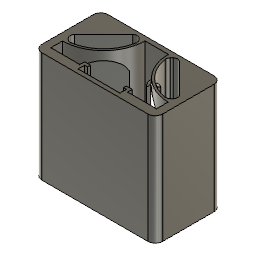
Imaging_Enclosure (Autodesk Fusion 360 design; units mm, degrees)
part number: 2026-03-22-21-42-42-827
Autodesk Fusion 360 part; units mm, degrees
note: some values were not read from the file. Set by a fixed rule: which face or edge a step refers to.
sketch "Sketch1" plane through (0, 0, 0) normal (0, 0, 1) x (1, 0, 0)
  line L0 (-43.0895, 22.8761) -> (56.9105, 22.8761)
  line L1 (56.9105, 22.8761) -> (56.9105, -20.1239)
  line L2 (56.9105, -20.1239) -> (-43.0895, -20.1239)
  line L3 (-43.0895, -20.1239) -> (-43.0895, 22.8761)
  dimension "d1" = 100
  dimension "d2" = 43
  constraint horizontal L0
  constraint vertical L1
  constraint horizontal L2
  constraint vertical L3
  measures "d1" distance of L0.start L0.end
  measures "d2" distance of L0.start L2.end
extrude "Extrude1" add sketch "Sketch1" along normal blind 75 makes body 1
sketch "TOP" plane through (0, 0, 75) normal (0, 0, 1) x (-1, 0, 0)
  line L0 (43.0895, 20.1239) -> (-56.9105, 20.1239)
  line L1 (-56.9105, 20.1239) -> (-56.9105, -22.8761)
  line L2 (-56.9105, -22.8761) -> (43.0895, -22.8761)
  line L3 (43.0895, -22.8761) -> (43.0895, 20.1239)
  line L4 (39.0895, -19.8761) -> (-52.9105, -19.8761)
  line L5 (-52.9105, -19.8761) -> (-52.9105, 16.1239)
  line L6 (-52.9105, 16.1239) -> (39.0895, 16.1239)
  line L7 (39.0895, 16.1239) -> (39.0895, -19.8761)
  line L8 (-6.9105, 16.1239) -> (-6.9105, 19.1239)
  line L9 (-6.9105, 16.1239) -> (16.0704, -6.8571)
  line L10 (-6.9105, 16.1239) -> (25.5895, 16.1239) construction
  line L11 (-6.9105, 16.1239) -> (-32.3664, -9.332)
  line L12 (-6.9105, 16.1239) -> (29.0895, 16.1239) construction
  line L13 (-32.3664, -9.332) -> (-21.8222, -19.8761)
  line L14 (-32.3664, -9.332) -> (-17.4547, -9.332) construction
  line L15 (-32.3664, -9.332) -> (-52.9105, 11.2122)
  line L16 (16.0704, -6.8571) -> (3.0514, -19.8761)
  line L17 (16.0704, -6.8571) -> (39.0895, 16.1619)
  line L18 (16.0704, -6.8571) -> (48.6243, -6.8571) construction
  line L19 (-32.3664, -9.332) -> (-44.2281, 2.5297)
  line L20 (-32.3664, -9.332) -> (-15.5914, -9.332) construction
  line L21 (-32.3664, -9.332) -> (-20.5047, -21.1937)
  line L22 (-20.5047, -21.1937) -> (-16.501, -17.1901)
  line L23 (-20.5047, -21.1937) -> (-14.8427, -21.1937) construction
  line L24 (-44.2281, 2.5297) -> (-40.2245, 6.5334)
  line L25 (-32.3664, -9.332) -> (-24.1993, -1.1649)
  line L26 (-20.5047, -21.1937) -> (-19.0904, -19.7795)
  line L27 (-19.0904, -19.7795) -> (-16.3404, -19.7795)
  line L28 (-44.2281, 2.5297) -> (-42.8139, 3.9439)
  line L29 (-42.8139, 3.9439) -> (-42.8139, 6.6939)
  arc A0 (-16.3404, -19.7795) -> (-42.8139, 6.6939) centre (-43.1782, -20.1438) ccw
  line L30 (-24.1993, -1.1649) -> (-23.1386, -0.1042)
  line L31 (-16.3404, -19.7795) -> (-14.8404, -19.7795)
  line L32 (-42.8139, 6.6939) -> (-42.8139, 8.1939)
  line L33 (-42.8139, 8.1939) -> (-42.8139, 16.1239)
  arc A1 (-14.8404, -19.7795) -> (-42.8139, 8.1939) centre (-43.1779, -20.1435) ccw
  line L34 (-6.9105, 16.1239) -> (-6.9105, -19.8761)
  line L35 (-16.501, -17.1901) -> (-20.5047, -21.1937)
  line L36 (-40.2245, 6.5334) -> (-44.2281, 2.5297)
  line L37 (-40.2245, 6.5334) -> (-44.2281, 2.5297)
  line L38 (-42.8139, 3.9439) -> (-40.2245, 6.5334)
  line L39 (-19.1871, -19.8761) -> (-16.501, -17.1901)
  line L40 (-24.1993, -1.1649) -> (-32.6492, -9.6148)
  line L41 (-32.6492, -9.6148) -> (-20.6461, -21.618)
  line L42 (-32.6492, -9.6148) -> (-15.6742, -9.6148) construction
  line L43 (-20.6461, -21.618) -> (-16.4739, -17.4458)
  line L44 (-32.6492, -9.6148) -> (-44.6524, 2.3883)
  line L45 (-32.6492, -9.6148) -> (-15.6742, -9.6148) construction
  line L46 (-44.6524, 2.3883) -> (-40.4802, 6.5605)
  line L47 (-14.8404, -19.7795) -> (-14.8404, -19.8761)
  line L48 (7.2891, 14.9239) -> (-21.1109, 14.9239)
  line L49 (-21.1109, 14.9239) -> (-21.1109, 19.3239)
  line L50 (-21.1109, 19.3239) -> (7.2891, 19.3239)
  line L51 (7.2891, 19.3239) -> (7.2891, 14.9239)
  line L52 (-6.9105, 16.1239) -> (0.1895, 16.1239)
  dimension "d5" = 92
  dimension "d6" = 36
  dimension "d7" = 4
  dimension "d8" = 3
  dimension "d9" = 3
  dimension "d10" = 46
  dimension "d11" = 32.5
  dimension "d12" = 45
  dimension "d13" = 135
  dimension "d14" = 36
  dimension "d15" = 45
  dimension "d16" = 45
  dimension "d17" = 135
  dimension "d18" = 16.775
  dimension "d19" = 16.775
  dimension "d20" = 45
  dimension "d21" = 5.662
  dimension "d22" = 5.662
  dimension "d23" = 11.55
  dimension "d24" = 2
  dimension "d25" = 2.75
  dimension "d26" = 2
  dimension "d27" = 2.75
  dimension "d28" = 1.5
  dimension "d29" = 1.5
  dimension "d30" = 1.5
  dimension "d31" = 11.95
  dimension "d32" = 45
  dimension "d33" = 16.975
  dimension "d34" = 135
  dimension "d35" = 16.975
  dimension "d105" = 28.4
  dimension "d106" = 4.4
  dimension "d107" = 1.2
  dimension "d108" = 21.703
  dimension "d124" = 7.1
  constraint horizontal L4
  constraint vertical L5
  constraint horizontal L6
  constraint vertical L7
  constraint coincident L6 L8.start
  constraint perpendicular L6 L8
  constraint horizontal L10
  constraint horizontal L12
  constraint horizontal L14
  constraint coincident L4 L13.end
  constraint coincident L5 L15.end
  constraint perpendicular L11 L15
  constraint coincident L4 L16.end
  constraint perpendicular L9 L16
  constraint horizontal L18
  constraint coincident L7 L17.end
  constraint horizontal L20
  constraint perpendicular L11 L21
  constraint horizontal L23
  constraint perpendicular L19 L24
  constraint perpendicular L13 L25
  constraint perpendicular L21 L26
  constraint horizontal L27
  constraint perpendicular L19 L28
  constraint vertical L29
  constraint coincident L25.end A0
  constraint parallel L11 L30
  constraint parallel L27 L31
  constraint parallel L29 L32
  constraint vertical L33
  constraint coincident L6 L33.end
  constraint coincident L30.end A1
  constraint midpoint L4 L34.end
  constraint coincident L4 L39.start
  constraint coincident L26 L39.start
  constraint parallel L25 L40
  constraint horizontal L42
  constraint coincident A0 L43.end
  constraint perpendicular L41 L43
  constraint horizontal L45
  constraint coincident A0 L46.end
  constraint perpendicular L44 L46
  constraint vertical L47
  constraint coincident L4 L47.end
  constraint horizontal L48
  constraint vertical L49
  constraint horizontal L50
  constraint vertical L51
  constraint perpendicular L51 L52
  measures "d5" distance of L4.start L4.end
  measures "d6" distance of L4.start L6.end
  measures "d7" distance of L1 L5
  measures "d8" distance of L2 L4
  measures "d9" distance of L8.start L8.end
  measures "d10" distance of L5 L8
  measures "d11" distance of L8.start L9.end
  measures "d12" angle of L9 L10
  measures "d13" angle of L11 L12
  measures "d14" distance of L8.start L11.end
  measures "d15" angle of L13 L14
  measures "d16" angle of L17 L18
  measures "d17" angle of L19 L20
  measures "d18" distance of L11.end L19.end
  measures "d19" distance of L11.end L21.end
  measures "d20" angle of L22 L23
  measures "d21" distance of L21.end L22.end
  measures "d22" distance of L19.end L24.end
  measures "d23" distance of L11.end L25.end
  measures "d24" distance of L21.end L26.end
  measures "d25" distance of L26.end L27.end
  measures "d26" distance of L19.end L28.end
  measures "d27" distance of L28.end L29.end
  measures "d28" distance of L25.end L30.end
  measures "d29" distance of L27.end L31.end
  measures "d30" distance of L29.end L32.end
  measures "d31" distance of L25.end L40.end
  measures "d32" angle of L41 L42
  measures "d33" distance of L40.end L41.end
  measures "d34" angle of L44 L45
  measures "d35" distance of L40.end L44.end
  measures "d105" distance of L48.start L48.end
  measures "d106" distance of L48.start L50.end
  measures "d107" distance of L12 L48
  measures "d108" distance of L33 L49
  measures "d124" distance of L8.start L52.end
sketch "Sketch3" plane through (0, -20.1239, 0) normal (0, -1, 0) x (1, 0, 0)
  line L0 (-43.0895, 0) -> (56.9105, 0)
  line L1 (56.9105, 0) -> (56.9105, 75)
  line L2 (56.9105, 75) -> (-43.0895, 75)
  line L3 (-43.0895, 75) -> (-43.0895, 0)
extrude "Extrude2" cut sketch "TOP" against normal blind 41.25 contours L4 L21 L22 L26 L35 L41 L43 | L4 L22 L26 L27 L35 L39 L43 | L4 L21 L22 L26 L35 | L4 L11 L13 L21 L22 L25 L26 A0 L35 L39 L40 | L22 L27 A0 L35 L39 L43 | L4 L13 L21 L40 L41 | L11 L15 L19 L24 L25 L28 A0 L36 L37 L38 L40 | L15 L19 L40 L44 L46 | L24 L29 A0 L36 L37 L38 L46 | L15 L24 L28 L29 L36 L37 L46 bodies 1
extrude "Extrude3" cut sketch "TOP" against normal blind 51.25 contours L4 L21 L22 L26 L35 L41 L43 | L4 L22 L26 L27 L35 L39 L43 | L4 L21 L22 L26 L35 | L4 L11 L13 L21 L22 L25 L26 A0 L35 L39 L40 | L22 L27 A0 L35 L39 L43 | L4 L13 L21 L40 L41 | L11 L15 L19 L24 L25 L28 A0 L36 L37 L38 L40 | L15 L19 L40 L44 L46 | L24 L29 A0 L36 L37 L38 L46 | L15 L24 L28 L29 L36 L37 L46 bodies 1
extrude "Extrude4" cut sketch "TOP" against normal blind 71 contours L4 L9 L16 L34 L48 | L4 L11 A1 L34 L47 L48 | L6 L9 L17 L48 L51 | L11 L34 L48 | L9 L34 L48 | L6 L9 L48 L51 L52 | L6 L11 L48 L49 | L6 L11 L33 A1 L48 L49 bodies 1
sketch "Sketch4" plane through (21.132, 21.132, 0) normal (-0.707107, -0.707107, 0) x (0.707107, -0.707107, 0)
  line L0 (33.2628, 75) -> (-0.6872, 75)
  line L1 (-0.6872, 75) -> (-0.6872, 23.75)
  line L2 (-0.6872, 23.75) -> (33.2628, 23.75)
  line L3 (33.2628, 23.75) -> (33.2628, 75)
  line L4 (3.9498, 60.75) -> (28.6258, 60.75)
  line L5 (28.6258, 60.75) -> (28.6258, 27.75)
  line L6 (28.6258, 27.75) -> (3.9498, 27.75)
  line L7 (3.9498, 27.75) -> (3.9498, 60.75)
  line L8 (3.9498, 54.2255) -> (16.2878, 54.2255) construction
  line L9 (16.2878, 54.2255) -> (16.2878, 27.75) construction
  line L10 (16.2878, 54.2255) -> (16.2878, 68.7495) construction
  arc A0 (28.6258, 60.75) -> (3.9498, 60.75) centre (16.2878, 55.2351) ccw construction
  dimension "d42" = 24.676
  dimension "d43" = 33
  dimension "d44" = 4.637
  dimension "d45" = 4
  dimension "d46" = 12.338
  dimension "d47" = 14.524
  constraint horizontal L4
  constraint vertical L5
  constraint horizontal L6
  constraint vertical L7
  constraint coincident L7 L8.start
  constraint perpendicular L7 L8
  constraint midpoint L6 L9.end
  constraint perpendicular L8 L10
  constraint coincident L10.end A0
  measures "d42" distance of L4.start L4.end
  measures "d43" distance of L4.start L6.end
  measures "d44" distance of L1 L7
  measures "d45" distance of L2 L6
  measures "d46" distance of L8.start L8.end
  measures "d47" distance of L8.end L10.end
sketch "Sketch5" plane through (21.132, 21.132, 0) normal (-0.707107, -0.707107, 0) x (0.707107, -0.707107, 0)
  line L0 (33.2628, 75) -> (-0.6872, 75)
  line L1 (-0.6872, 75) -> (-0.6872, 23.75)
  line L2 (-0.6872, 23.75) -> (33.2628, 23.75)
  line L3 (33.2628, 23.75) -> (33.2628, 75)
  line L4 (3.9498, 61.1) -> (28.6258, 61.1)
  line L5 (28.6258, 61.1) -> (28.6258, 28.1)
  line L6 (28.6258, 28.1) -> (3.9498, 28.1)
  line L7 (3.9498, 28.1) -> (3.9498, 61.1)
  line L8 (16.2878, 28.1) -> (16.2878, 69.1)
  arc A0 (28.6258, 61.1) -> (3.9498, 61.1) centre (16.2878, 55.5859) ccw
  dimension "d48" = 24.676
  dimension "d49" = 33
  dimension "d50" = 4.637
  dimension "d51" = 4.35
  dimension "d52" = 41
  constraint horizontal L4
  constraint vertical L5
  constraint horizontal L6
  constraint vertical L7
  constraint vertical L8
  constraint midpoint L6 L8.start
  constraint coincident L8.end A0
  measures "d48" distance of L4.start L4.end
  measures "d49" distance of L4.start L6.end
  measures "d50" distance of L1 L7
  measures "d51" distance of L2 L6
  measures "d52" distance of L8.start L8.end
extrude "Extrude5" cut sketch "Sketch5" along normal blind 14 contours L4 L8 A0 | L4 L6 L7 L8 | L4 L8 A0 | L4 L5 L6 L8 bodies 1
fillet "Fillet1" radius 3 4 edges at (20.6461, 21.618, 49.375) (16.4739, 17.4458, 49.375) (40.4802, -6.5605, 49.375) (44.6524, -2.3883, 49.375) on bodies 1
sketch "Sketch6" plane through (0, 22.8761, 0) normal (0, 1, 0) x (-1, 0, 0)
  line L0 (-56.9105, 0) -> (43.0895, 0)
  line L1 (43.0895, 0) -> (43.0895, 75)
  line L2 (43.0895, 75) -> (-56.9105, 75)
  line L3 (-56.9105, 75) -> (-56.9105, 0)
  line L4 (-6.9105, 0) -> (-6.9105, 75)
  line L5 (43.0895, 7.2495) -> (-56.9105, 7.2495)
  circle A0 centre (-6.9105, 35.85) radius 7
  circle A1 centre (-6.9105, 48.35) radius 7
  line L6 (3.5895, 23.35) -> (-17.4105, 23.35)
  line L7 (-17.4105, 23.35) -> (-17.4105, 35.85)
  line L8 (-17.4105, 35.85) -> (3.5895, 35.85)
  line L9 (3.5895, 35.85) -> (3.5895, 23.35)
  line L10 (3.5895, 35.85) -> (-17.4105, 35.85)
  line L11 (-17.4105, 35.85) -> (-17.4105, 48.35)
  line L12 (-17.4105, 48.35) -> (3.5895, 48.35)
  line L13 (3.5895, 48.35) -> (3.5895, 35.85)
  line L14 (3.5895, 29.6) -> (-17.4105, 29.6)
  line L15 (-17.4105, 29.6) -> (-17.4105, 42.1)
  line L16 (-17.4105, 42.1) -> (3.5895, 42.1)
  line L17 (3.5895, 42.1) -> (3.5895, 29.6)
  line L18 (0.0895, 48.35) -> (0.0895, 35.85)
  line L19 (-13.9105, 35.85) -> (-13.9105, 48.35)
  line L20 (-2.5605, 22.65) -> (-11.2605, 22.65)
  line L21 (-11.2605, 22.65) -> (-11.2605, 34.65)
  line L22 (-11.2605, 34.65) -> (-2.5605, 34.65)
  line L23 (-2.5605, 34.65) -> (-2.5605, 22.65)
  circle A2 centre (3.5895, 23.35) radius 0.85
  circle A3 centre (3.5895, 29.6) radius 0.85
  circle A4 centre (3.5895, 35.85) radius 0.85
  circle A5 centre (3.5895, 42.1) radius 0.85
  circle A6 centre (3.5895, 48.35) radius 0.85
  circle A7 centre (-17.4105, 48.35) radius 0.85
  circle A8 centre (-17.4105, 42.1) radius 0.85
  circle A9 centre (-17.4105, 35.85) radius 0.85
  circle A10 centre (-17.4105, 29.6) radius 0.85
  circle A11 centre (-17.4105, 23.35) radius 0.85
  dimension "d57" = 50
  dimension "d58" = 14
  dimension "d59" = 50
  dimension "d60" = 35.85
  dimension "d61" = 14
  dimension "d62" = 48.35
  dimension "d72" = 21
  dimension "d73" = 12.5
  dimension "d74" = 12.5
  dimension "d75" = 10.5
  dimension "d76" = 21
  dimension "d77" = 12.5
  dimension "d78" = 12.5
  dimension "d79" = 10.5
  dimension "d80" = 21
  dimension "d81" = 12.5
  dimension "d82" = 6.25
  dimension "d83" = 8.7
  dimension "d84" = 12
  dimension "d85" = 0.7
  dimension "d86" = 4.35
  dimension "d87" = 1.7
  dimension "d88" = 1.7
  dimension "d89" = 1.7
  dimension "d90" = 1.7
  dimension "d91" = 1.7
  dimension "d92" = 1.7
  dimension "d93" = 1.7
  dimension "d94" = 1.7
  dimension "d95" = 1.7
  dimension "d96" = 1.7
  constraint coincident L0 L4.start
  constraint coincident L2 L4.end
  constraint perpendicular L2 L4
  constraint coincident L1 L5.start
  constraint coincident L3 L5.end
  constraint perpendicular L3 L5
  constraint coincident L4 A1.centre
  constraint horizontal L6
  constraint vertical L7
  constraint horizontal L8
  constraint vertical L9
  constraint horizontal L10
  constraint vertical L11
  constraint horizontal L12
  constraint vertical L13
  constraint horizontal L14
  constraint vertical L15
  constraint horizontal L16
  constraint vertical L17
  constraint coincident L9 L14.start
  constraint coincident L12 L18.start
  constraint coincident A1 L18.start
  constraint coincident L10 L18.end
  constraint coincident A0 L18.end
  constraint coincident A0 L19.start
  constraint coincident L8 L19.start
  constraint coincident A1 L19.end
  constraint coincident L12 L19.end
  constraint horizontal L20
  constraint vertical L21
  constraint horizontal L22
  constraint vertical L23
  constraint coincident L6.start L9.end
  constraint coincident L14.start L17.end
  constraint coincident L8.end L9.start
  constraint coincident L16.end L17.start
  constraint coincident L12.end L13.start
  constraint coincident L11.end L12.start
  constraint coincident L15.end L16.start
  constraint coincident L7.end L8.start
  constraint coincident L14.end L15.start
  constraint coincident L6.end L7.start
  measures "d57" distance of L3 L4
  measures "d58" diameter of A0
  measures "d59" distance of L3 A0.centre
  measures "d60" distance of L0 A0.centre
  measures "d61" diameter of A1
  measures "d62" distance of L0 A1.centre
  measures "d72" distance of L6.start L6.end
  measures "d73" distance of L6.start L8.end
  measures "d74" distance of A0.centre L6
  measures "d75" distance of A0.centre L7
  measures "d76" distance of L8.end L7.end
  measures "d77" distance of L8.end L12.end
  measures "d78" distance of A1.centre L10
  measures "d79" distance of A1.centre L11
  measures "d80" distance of L14.start L14.end
  measures "d81" distance of L14.start L16.end
  measures "d82" distance of L12 L16
  measures "d83" distance of L20.start L20.end
  measures "d84" distance of L20.start L22.end
  measures "d85" distance of L6 L20
  measures "d86" distance of L4 L21
  measures "d87" diameter of A2
  measures "d88" diameter of A3
  measures "d89" diameter of A4
  measures "d90" diameter of A5
  measures "d91" diameter of A6
  measures "d92" diameter of A7
  measures "d93" diameter of A8
  measures "d94" diameter of A9
  measures "d95" diameter of A10
  measures "d96" diameter of A11
extrude "Extrude6" add 1 faces at (17.6517, 10.4832, 28.1) along direction (0, 0, 1) blind 45 on bodies 1 bodies 1
extrude "Extrude7" add 1 faces at (29.408, 7.2534, 23.75) along direction (0, 0, 1) blind 0.35 on bodies 1 bodies 1
extrude "Extrude8" cut sketch "Sketch5" along normal blind 15 contours L4 L8 A0 | L4 L6 L7 L8 | L4 L8 A0 | L4 L5 L6 L8 bodies 1
sketch "Sketch7" plane through (0, 0, 0) normal (0, 1, 0) x (1, 0, 0)
extrude "Extrude9" cut sketch "Sketch6" against normal blind 2.5 contours L6 L9 A2 | L6 L9 A2 | L6 L7 A11 | L6 L7 A11 | L12 L13 A6 | L12 L13 A6 | L11 L12 A7 | L11 L12 A7 | L9 L14 L17 A3 | L9 L14 A3 | L7 L14 A10 | L7 L14 L15 A10 | L13 L16 A5 | L13 L16 L17 A5 | L11 L15 L16 A8 | L11 L16 A8 | L9 L17 A3 | L7 L15 A10 | L8 L10 L13 L17 A4 | L8 L9 L10 L17 A4 | L13 L17 A5 | L7 L8 L10 L15 A9 | L8 L10 L11 L15 A9 | L11 L15 A8 | L9 L13 L17 A4 | L7 L11 L15 A9 bodies 1
extrude "Extrude10" cut sketch "Sketch6" against normal blind 3 contours L4 L6 L20 L21 | L4 L6 L20 L23 | L4 A0 L6 L14 L21 | L4 A0 L6 L14 L23 | L4 A1 L12 | L4 A1 L12 | L4 A0 L14 | L4 A0 L14 | L4 A0 A1 L12 | L4 A0 A1 L12 | A1 L16 L18 | A1 L16 L19 | L4 A0 L14 L21 L22 | L4 A0 L14 L22 L23 | A0 L14 L21 | A0 L14 L23 | L4 A0 L16 | L4 A0 L16 | A0 L16 L18 | L4 A0 A1 L8 L10 | L4 A1 L16 | L4 A0 A1 L8 L10 | L4 A1 L16 | A0 L16 L19 | L4 A0 L8 L10 L21 L22 | L4 A0 L8 L10 L22 L23 bodies 1
sketch "Sketch8" plane through (0, 0, 4) normal (0, 0, 1) x (-1, 0, 0)
  arc A0 (-14.8404, -19.7795) -> (-42.8139, 8.1939) centre (-43.1779, -20.1435) ccw
  line L0 (-14.8404, -19.7795) -> (-14.8404, -19.8761)
  line L1 (-14.8404, -19.8761) -> (3.0514, -19.8761)
  line L2 (3.0514, -19.8761) -> (39.0514, 16.1239)
  line L3 (39.0514, 16.1239) -> (-42.8139, 16.1239)
  line L4 (-42.8139, 16.1239) -> (-42.8139, 8.1939)
  line L5 (7.2891, 14.9239) -> (-21.1109, 14.9239)
  line L6 (-21.1109, 14.9239) -> (-21.1109, 19.3239)
  line L7 (-21.1109, 19.3239) -> (7.2891, 19.3239)
  line L8 (7.2891, 19.3239) -> (7.2891, 14.9239)
  dimension "d101" = 28.4
  dimension "d102" = 4.4
  dimension "d103" = 1.2
  dimension "d104" = 21.703
  constraint horizontal L5
  constraint vertical L6
  constraint horizontal L7
  constraint vertical L8
  measures "d101" distance of L5.start L5.end
  measures "d102" distance of L5.start L7.end
  measures "d103" distance of L3 L5
  measures "d104" distance of L4 L6
extrude "Extrude11" cut sketch "TOP" against normal blind 75 contours L11 L34 L48 | L9 L34 L48 | L6 L9 L48 L51 L52 | L6 L49 L50 L51 L52 | L6 L11 L48 L49 bodies 1
extrude "Extrude12" add 1 faces at (23.5772, -20.1239, 25) along direction (0, -1, 0) blind 2 on bodies 1 bodies 1
sketch "Sketch9" plane through (0, 0, 75) normal (0, 0, 1) x (-1, 0, 0)
  line L0 (-56.9105, 22.1239) -> (-56.9105, -22.8761)
  line L1 (-56.9105, -22.8761) -> (43.0895, -22.8761)
  line L2 (43.0895, -22.8761) -> (43.0895, 22.1239)
  line L3 (43.0895, 22.1239) -> (-56.9105, 22.1239)
  line L4 (-17.5175, -18.4894) -> (-18.5248, -19.4967)
  arc A0 (-22.7674, -19.4967) -> (-18.5248, -19.4967) centre (-20.6461, -17.3753) ccw
  line L5 (-22.7674, -19.4967) -> (-42.531, 0.267)
  arc A1 (-42.531, 4.5096) -> (-42.531, 0.267) centre (-40.4097, 2.3883) ccw
  line L6 (-42.531, 4.5096) -> (-41.5238, 5.5168)
  arc A2 (-38.9274, 6.3577) -> (-41.5238, 5.5168) centre (-39.4025, 3.3955) ccw
  arc A3 (-16.6767, -15.893) -> (-38.9274, 6.3577) centre (-43.1782, -20.1438) ccw
  arc A4 (-17.5175, -18.4894) -> (-16.6767, -15.893) centre (-19.6389, -16.3681) ccw
  line L7 (-21.1109, 16.1239) -> (-21.1109, 19.3239)
  line L8 (-21.1109, 19.3239) -> (7.2891, 19.3239)
  line L9 (7.2891, 19.3239) -> (7.2891, 16.1239)
  line L10 (7.2891, 16.1239) -> (39.0514, 16.1239)
  line L11 (39.0514, 16.1239) -> (3.0514, -19.8761)
  line L12 (3.0514, -19.8761) -> (-14.8404, -19.8761)
  line L13 (-14.8404, -19.8761) -> (-14.8404, -19.7795)
  arc A5 (-14.8404, -19.7795) -> (-42.8139, 8.1939) centre (-43.1779, -20.1435) ccw
  line L14 (-42.8139, 8.1939) -> (-42.8139, 16.1239)
  line L15 (-42.8139, 16.1239) -> (-21.1109, 16.1239)
  line L16 (20.0558, 22.1239) -> (-47.9442, 22.1239)
  line L17 (-47.9442, 22.1239) -> (-47.9442, -22.8761)
  line L18 (-47.9442, -22.8761) -> (20.0558, -22.8761)
  line L19 (20.0558, -22.8761) -> (20.0558, 22.1239)
  line L20 (20.0558, 22.1239) -> (23.0558, 22.1239)
  line L21 (23.0558, 22.1239) -> (23.0558, -22.8761)
  dimension "d113" = 68
  dimension "d116" = 3
  constraint horizontal L16
  constraint vertical L17
  constraint horizontal L18
  constraint vertical L19
  constraint coincident L3 L16.start
  constraint perpendicular L19 L20
  constraint coincident L1 L21.end
  constraint perpendicular L1 L21
  measures "d113" distance of L16.start L16.end
  measures "d116" distance of L16.start L20.end
extrude "Extrude13" cut sketch "Sketch9" against normal blind 75 contours L0 L1 L3 L17 bodies 1
extrude "Extrude14" add sketch "Sketch9" against normal blind 75 contours L3 L10 L19 L20 L21 | L1 L11 L19 L21 | L10 L11 L19 L21 bodies 1
extrude "Extrude15" cut sketch "Sketch9" against normal blind 75 contours L1 L2 L3 L10 L11 L21 | L10 L11 L21 bodies 1
sketch "Sketch10" plane through (0, -14.9239, 0) normal (0, -1, 0) x (1, 0, 0)
  line L0 (21.1109, 4) -> (-7.2891, 4)
  line L1 (-7.2891, 4) -> (-7.2891, 0)
  line L2 (-7.2891, 0) -> (21.1109, 0)
  line L3 (21.1109, 0) -> (21.1109, 4)
chamfer "Chamfer1" distance 4 angle 45 1 edges at (6.9109, -14.9239, 0) on bodies 1
sketch "Sketch11" plane through (0, 22.8761, 0) normal (0, 1, 0) x (-1, 0, 0)
  arc A0 (-2.5605, 30.3657) -> (0.0895, 35.85) centre (-6.9105, 35.85) ccw
  line L0 (-2.5605, 30.3657) -> (-2.5605, 22.65)
  line L1 (-2.5605, 22.65) -> (-11.2605, 22.65)
  line L2 (-11.2605, 22.65) -> (-11.2605, 30.3657)
  arc A1 (-13.9105, 35.85) -> (-11.2605, 30.3657) centre (-6.9105, 35.85) ccw
  line L3 (-13.9105, 35.85) -> (-13.9105, 48.35)
  arc A2 (0.0895, 48.35) -> (-13.9105, 48.35) centre (-6.9105, 48.35) ccw
  line L4 (0.0895, 48.35) -> (0.0895, 35.85)
  circle A3 centre (3.5895, 29.6) radius 0.85
  circle A4 centre (-17.4105, 48.35) radius 0.85
  circle A5 centre (-17.4105, 29.6) radius 0.85
  circle A6 centre (3.5895, 48.35) radius 0.85
  circle A7 centre (3.5895, 23.35) radius 0.85
  circle A8 centre (3.5895, 35.85) radius 0.85
  circle A9 centre (-17.4105, 42.1) radius 0.85
  circle A10 centre (-17.4105, 35.85) radius 0.85
  circle A11 centre (3.5895, 42.1) radius 0.85
  circle A12 centre (-17.4105, 23.35) radius 0.85
  line L5 (23.0558, 75) -> (-47.9442, 75)
  line L6 (-47.9442, 0) -> (23.0558, 0)
  line L7 (23.0558, 0) -> (23.0558, 75)
  line L8 (-47.9442, 75) -> (-47.9442, 0)
sketch "Sketch12" plane through (0, 0, 75) normal (0, 0, 1) x (-1, 0, 0)
  line L0 (-48, 22) -> (-7, 22)
  constraint horizontal L0
sketch "Sketch13" plane through (0, 0, 75) normal (0, 0, 1) x (-1, 0, 0)
  line L0 (-17.5175, -18.4894) -> (-18.5248, -19.4967)
  arc A0 (-22.7674, -19.4967) -> (-18.5248, -19.4967) centre (-20.6461, -17.3753) ccw
  line L1 (-22.7674, -19.4967) -> (-42.531, 0.267)
  arc A1 (-42.531, 4.5096) -> (-42.531, 0.267) centre (-40.4097, 2.3883) ccw
  line L2 (-42.531, 4.5096) -> (-41.5238, 5.5168)
  arc A2 (-38.9274, 6.3577) -> (-41.5238, 5.5168) centre (-39.4025, 3.3955) ccw
  arc A3 (-16.6767, -15.893) -> (-38.9274, 6.3577) centre (-43.1782, -20.1438) ccw
  arc A4 (-17.5175, -18.4894) -> (-16.6767, -15.893) centre (-19.6389, -16.3681) ccw
  line L3 (20.0558, 16.1239) -> (20.0558, -2.8718)
  line L4 (20.0558, -2.8718) -> (3.0514, -19.8761)
  line L5 (3.0514, -19.8761) -> (-14.8404, -19.8761)
  line L6 (-14.8404, -19.8761) -> (-14.8404, -19.7795)
  arc A5 (-14.8404, -19.7795) -> (-42.8139, 8.1939) centre (-43.1779, -20.1435) ccw
  line L7 (-42.8139, 8.1939) -> (-42.8139, 16.1239)
  line L8 (-42.8139, 16.1239) -> (-21.1109, 16.1239)
  line L9 (-21.1109, 16.1239) -> (-21.1109, 19.3239)
  line L10 (-21.1109, 19.3239) -> (7.2891, 19.3239)
  line L11 (7.2891, 19.3239) -> (7.2891, 16.1239)
  line L12 (7.2891, 16.1239) -> (20.0558, 16.1239)
  line L13 (23.0558, -22.8761) -> (23.0558, 22.1239)
  line L14 (23.0558, 22.1239) -> (-47.9442, 22.1239)
  line L15 (-47.9442, 22.1239) -> (-47.9442, -22.8761)
  line L16 (-47.9442, -22.8761) -> (23.0558, -22.8761)
  line L17 (-21.1109, 22.1239) -> (-47.9442, 22.1239)
  line L18 (7.2891, 19.3239) -> (-21.1109, 19.3239)
  line L19 (-21.1109, 19.3239) -> (-6.9109, 19.3239)
  line L20 (-21.1109, 19.3239) -> (-47.9442, 19.3239)
  line L21 (-6.9109, 19.3239) -> (-47.9442, 19.3239)
  dimension "d129" = 14.2
  constraint coincident L14 L17.start
  constraint coincident L14.end L15.start
  constraint coincident L10.end L11.start
  constraint coincident L9.end L10.start
  constraint coincident L15 L20.end
  constraint perpendicular L15 L20
  constraint perpendicular L15 L21
  measures "d129" distance of L9.end L19.end
sketch "Sketch14" plane through (0, 22.8761, 0) normal (0, 1, 0) x (-1, 0, 0)
  line L0 (23.0558, 0) -> (23.0558, 75)
  line L1 (23.0558, 75) -> (-47.9442, 75)
  line L2 (-47.9442, 75) -> (-47.9442, 0)
  line L3 (-47.9442, 0) -> (23.0558, 0)
  circle A0 centre (-17.4105, 23.35) radius 0.85
  circle A1 centre (3.5895, 42.1) radius 0.85
  circle A2 centre (-17.4105, 35.85) radius 0.85
  circle A3 centre (-17.4105, 42.1) radius 0.85
  circle A4 centre (3.5895, 35.85) radius 0.85
  circle A5 centre (3.5895, 23.35) radius 0.85
  circle A6 centre (3.5895, 48.35) radius 0.85
  circle A7 centre (-17.4105, 29.6) radius 0.85
  circle A8 centre (-17.4105, 48.35) radius 0.85
  circle A9 centre (3.5895, 29.6) radius 0.85
  arc A10 (-2.5605, 30.3657) -> (0.0895, 35.85) centre (-6.9105, 35.85) ccw
  line L4 (-2.5605, 30.3657) -> (-2.5605, 22.65)
  line L5 (-2.5605, 22.65) -> (-11.2605, 22.65)
  line L6 (-11.2605, 22.65) -> (-11.2605, 30.3657)
  arc A11 (-13.9105, 35.85) -> (-11.2605, 30.3657) centre (-6.9105, 35.85) ccw
  line L7 (-13.9105, 35.85) -> (-13.9105, 48.35)
  arc A12 (0.0895, 48.35) -> (-13.9105, 48.35) centre (-6.9105, 48.35) ccw
  line L8 (0.0895, 48.35) -> (0.0895, 35.85)
  line L9 (-2.5605, 22.65) -> (-11.2605, 22.65)
  line L10 (-2.5605, 22.65) -> (-11.2605, 22.65)
  line L11 (-11.2605, 22.65) -> (-6.9105, 22.65)
  line L12 (-6.9105, 22.65) -> (-47.9442, 22.65)
  dimension "d128" = 4.35
  constraint coincident L4.end L5.start
  constraint coincident L5.end L6.start
  constraint perpendicular L6 L11
  constraint horizontal L12
  constraint coincident L2 L12.end
  measures "d128" distance of L5.end L11.end
ref_plane "WorkPlane2" through (6.9107, 0.3761, 37.5) normal (1, 0, 0) x (0, -1, 0)
split "Split1" by plane through (6.9107, 0.3761, 37.5) normal (1, 0, 0) bodies 1 makes body 2 at (47.9442, -7.1239, 50)
mirror "Mirror1" about plane through (6.9107, 0.3761, 37.5) normal (1, 0, 0) of bodies 2 merged
sketch "Sketch15" plane through (0, 0, 75) normal (0, 0, 1) x (-1, 0, 0)
sketch "Sketch16" plane through (0, 0, 75) normal (0, 0, 1) x (-1, 0, 0)
  line L0 (1.019, -19.8761) -> (-14.8404, -19.8761)
  line L1 (-14.8404, -19.8761) -> (-14.8404, -19.7795)
  arc A0 (-14.8404, -19.7795) -> (-42.8139, 8.1939) centre (-43.1779, -20.1435) ccw
  line L2 (-42.8139, 8.1939) -> (-42.8139, 16.1239)
  line L3 (-42.8139, 16.1239) -> (-21.1109, 16.1239)
  line L4 (-21.1109, 16.1239) -> (-21.1109, 19.3239)
  line L5 (-21.1109, 19.3239) -> (7.2894, 19.3239)
  line L6 (7.2894, 19.3239) -> (7.2894, 16.1239)
  line L7 (7.2894, 16.1239) -> (28.9924, 16.1239)
  line L8 (28.9924, 16.1239) -> (28.9924, 8.1939)
  arc A1 (28.9924, 8.1939) -> (1.019, -19.7795) centre (29.3564, -20.1435) ccw
  line L9 (1.019, -19.7795) -> (1.019, -19.8761)
  line L10 (4.7033, -19.4967) -> (3.6961, -18.4894)
  arc A2 (2.8553, -15.893) -> (3.6961, -18.4894) centre (5.8174, -16.3681) ccw
  arc A3 (25.1059, 6.3577) -> (2.8553, -15.893) centre (29.3567, -20.1438) ccw
  arc A4 (27.7024, 5.5168) -> (25.1059, 6.3577) centre (25.581, 3.3955) ccw
  line L11 (27.7024, 5.5168) -> (28.7096, 4.5096)
  arc A5 (28.7096, 0.267) -> (28.7096, 4.5096) centre (26.5883, 2.3883) ccw
  line L12 (28.7096, 0.267) -> (8.9459, -19.4967)
  arc A6 (4.7033, -19.4967) -> (8.9459, -19.4967) centre (6.8246, -17.3753) ccw
  line L13 (-47.9442, -22.8761) -> (34.1228, -22.8761)
  line L14 (34.1228, -22.8761) -> (34.1228, 22.1239)
  line L15 (34.1228, 22.1239) -> (-47.9442, 22.1239)
  line L16 (-47.9442, 22.1239) -> (-47.9442, -22.8761)
  line L17 (-17.5175, -18.4894) -> (-18.5248, -19.4967)
  arc A7 (-22.7674, -19.4967) -> (-18.5248, -19.4967) centre (-20.6461, -17.3753) ccw
  line L18 (-22.7674, -19.4967) -> (-42.531, 0.267)
  arc A8 (-42.531, 4.5096) -> (-42.531, 0.267) centre (-40.4097, 2.3883) ccw
  line L19 (-42.531, 4.5096) -> (-41.5238, 5.5168)
  arc A9 (-38.9274, 6.3577) -> (-41.5238, 5.5168) centre (-39.4025, 3.3955) ccw
  arc A10 (-16.6767, -15.893) -> (-38.9274, 6.3577) centre (-43.1782, -20.1438) ccw
  arc A11 (-17.5175, -18.4894) -> (-16.6767, -15.893) centre (-19.6389, -16.3681) ccw
  line L20 (7.2894, 19.3239) -> (-21.1109, 19.3239)
  constraint coincident L5.end L6.start
  constraint coincident L4.end L5.start
sketch "Sketch17" plane through (0, 22.8761, 0) normal (0, 1, 0) x (-1, 0, 0)
  line L0 (-2.5609, 22.65) -> (-11.2605, 22.65)
  line L1 (-11.2605, 22.65) -> (-11.2605, 30.3657)
  arc A0 (-13.9105, 35.85) -> (-11.2605, 30.3657) centre (-6.9105, 35.85) ccw
  line L2 (-13.9105, 35.85) -> (-13.9105, 48.35)
  arc A1 (-6.9107, 55.35) -> (-13.9105, 48.35) centre (-6.9105, 48.35) ccw
  arc A2 (0.0891, 48.35) -> (-6.9107, 55.35) centre (-6.9109, 48.35) ccw
  line L3 (0.0891, 48.35) -> (0.0891, 35.85)
  arc A3 (-2.5609, 30.3657) -> (0.0891, 35.85) centre (-6.9109, 35.85) ccw
  line L4 (-2.5609, 30.3657) -> (-2.5609, 22.65)
  circle A4 centre (3.5891, 48.35) radius 0.85
  circle A5 centre (3.5891, 29.6) radius 0.85
  circle A6 centre (3.5891, 42.1) radius 0.85
  circle A7 centre (3.5891, 35.85) radius 0.85
  circle A8 centre (3.5891, 23.35) radius 0.85
  line L5 (-47.9442, 0) -> (34.1228, 0)
  line L6 (34.1228, 0) -> (34.1228, 75)
  line L7 (34.1228, 75) -> (-47.9442, 75)
  line L8 (-47.9442, 75) -> (-47.9442, 0)
  circle A9 centre (-17.4105, 23.35) radius 0.85
  circle A10 centre (-17.4105, 35.85) radius 0.85
  circle A11 centre (-17.4105, 42.1) radius 0.85
  circle A12 centre (-17.4105, 29.6) radius 0.85
  circle A13 centre (-17.4105, 48.35) radius 0.85
  line L9 (-2.5609, 22.65) -> (-11.2605, 22.65)
  line L10 (3.5891, 23.35) -> (-17.4105, 23.35)
  line L11 (-17.4105, 23.35) -> (-17.4105, 35.85)
  constraint coincident L0.start L4.end
  constraint coincident L0.end L1.start
  constraint coincident A8.centre L10.start
  constraint coincident A9.centre L10.end
  constraint coincident A10.centre L11.end
sketch "Sketch18" plane through (0, 0, 0) normal (0, 0, -1) x (1, 0, 0)
  line L0 (-34.1228, -22.8761) -> (47.9442, -22.8761)
  line L1 (47.9442, -22.8761) -> (47.9442, 22.1239)
  line L2 (47.9442, 22.1239) -> (-34.1228, 22.1239)
  line L3 (-34.1228, 22.1239) -> (-34.1228, -22.8761)
  line L4 (21.1109, 10.9239) -> (-7.2894, 10.9239)
  line L5 (-7.2894, 10.9239) -> (-7.2894, 19.3239)
  line L6 (-7.2894, 19.3239) -> (21.1109, 19.3239)
  line L7 (21.1109, 19.3239) -> (21.1109, 10.9239)
  line L8 (10.9109, 19.3239) -> (2.9109, 19.3239)
  line L9 (2.9109, 19.3239) -> (2.9109, 11.8239)
  line L10 (2.9109, 11.8239) -> (10.9109, 11.8239)
  line L11 (10.9109, 11.8239) -> (10.9109, 19.3239)
  dimension "d133" = 8
  dimension "d134" = 7.5
  dimension "d135" = 10.2
  constraint horizontal L8
  constraint vertical L9
  constraint horizontal L10
  constraint vertical L11
  constraint coincident L6 L8.start
  measures "d133" distance of L8.start L8.end
  measures "d134" distance of L8.start L10.end
  measures "d135" distance of L7 L11
extrude "Extrude16" cut sketch "Sketch18" against normal blind 8 contours L6 L8 L9 L10 L11 bodies 2
fillet "Fillet3" radius 5 4 edges at (-34.1228, -22.1239, 37.5) (47.9442, -22.1239, 37.5) (47.9442, 22.8761, 37.5) (-34.1228, 22.8761, 37.5) on bodies 2
sketch "Sketch19" plane through (0, 0, 4) normal (0, 0, 1) x (-1, 0, 0)
  line L0 (-10.9109, 11.8239) -> (-10.9109, 14.9239)
  line L1 (-10.9109, 14.9239) -> (-21.1109, 14.9239)
  line L2 (-21.1109, 14.9239) -> (-21.1109, 16.1239)
  line L3 (-21.1109, 16.1239) -> (-42.8139, 16.1239)
  line L4 (-42.8139, 16.1239) -> (-42.8139, 8.1939)
  arc A0 (-14.8404, -19.7795) -> (-42.8139, 8.1939) centre (-43.1779, -20.1435) ccw
  line L5 (-14.8404, -19.7795) -> (-14.8404, -19.8761)
  line L6 (-14.8404, -19.8761) -> (1.019, -19.8761)
  line L7 (1.019, -19.8761) -> (1.019, -19.7795)
  arc A1 (28.9924, 8.1939) -> (1.019, -19.7795) centre (29.3564, -20.1435) ccw
  line L8 (28.9924, 8.1939) -> (28.9924, 16.1239)
  line L9 (28.9924, 16.1239) -> (7.2894, 16.1239)
  line L10 (7.2894, 16.1239) -> (7.2894, 14.9239)
  line L11 (7.2894, 14.9239) -> (-2.9109, 14.9239)
  line L12 (-2.9109, 14.9239) -> (-2.9109, 11.8239)
  line L13 (-2.9109, 11.8239) -> (-10.9109, 11.8239)
  line L14 (7.2894, 14.9239) -> (7.2894, 16.1239)
  line L15 (7.2894, 14.9239) -> (5.2894, 14.9239)
  line L16 (5.2894, 14.9239) -> (5.2894, 12.9239)
  line L17 (5.2894, 12.9239) -> (9.2894, 12.9239)
  line L18 (9.2894, 12.9239) -> (9.2894, 16.1239)
  line L19 (-21.1109, 16.1239) -> (-21.1109, 14.9239)
  line L20 (-21.1109, 14.9239) -> (-19.1109, 14.9239)
  line L21 (-19.1109, 14.9239) -> (-19.1109, 12.9239)
  line L22 (-19.1109, 12.9239) -> (-23.1109, 12.9239)
  line L23 (-23.1109, 12.9239) -> (-23.1109, 16.1239)
  dimension "d140" = 2
  dimension "d141" = 2
  dimension "d142" = 4
  dimension "d143" = 2
  dimension "d144" = 2
  dimension "d145" = 4
  constraint coincident L10.end L11.start
  constraint coincident L9.end L10.start
  constraint perpendicular L10 L15
  constraint perpendicular L11 L16
  constraint perpendicular L16 L17
  constraint coincident L9 L18.end
  constraint perpendicular L9 L18
  constraint coincident L2.end L3.start
  constraint coincident L1.end L2.start
  constraint perpendicular L2 L20
  constraint perpendicular L1 L21
  constraint perpendicular L21 L22
  constraint coincident L3 L23.end
  constraint perpendicular L3 L23
  measures "d140" distance of L10.end L15.end
  measures "d141" distance of L15.end L16.end
  measures "d142" distance of L16.end L17.end
  measures "d143" distance of L1.end L20.end
  measures "d144" distance of L20.end L21.end
  measures "d145" distance of L21.end L22.end
extrude "Extrude17" add sketch "Sketch19" along normal blind 50 contours L1 L2 L3 L19 L20 L21 L22 L23 | L9 L10 L11 L14 L15 L16 L17 L18 bodies 2
extrude "Extrude18" add 2 faces at (21.1109, -13.5905, 54) (-7.2894, -13.5905, 54) along direction (0, 0, 1) blind 30 on bodies 2 bodies 2
extrude "Extrude19" cut 2 faces at (21.7775, -16.1239, 81) (-8.6228, -16.1239, 81) along direction (0, 1, 0) blind 6 on bodies 2 bodies 2
extrude "Extrude20" cut 1 faces at (21.1109, -14.2572, 78) along direction (-1, 0, 0) blind 4 on bodies 2 bodies 2
extrude "Extrude21" cut 1 faces at (-7.2894, -14.2572, 78) along direction (1, 0, 0) blind 4 on bodies 2 bodies 2
extrude "Extrude22" cut 2 faces at (-15.5865, 7.2534, 24.1) (29.408, 7.2534, 24.1) along direction (0, 0, -1) blind 0.2 on bodies 2 bodies 2
hidden bodies 1
equation "d10 = ( 92 / 2 ) * 1 mm"
equation "d18 = ( 33.55 / 2 ) * 1 mm"
equation "d19 = ( 33.55 / 2 ) * 1 mm"
equation "d33 = ( 33.95 / 2 ) * 1 mm"
equation "d35 = ( 33.95 / 2 ) * 1 mm"
equation "d44 = ( ( 33.95 - 24.676 ) / 2 ) * 1 mm"
equation "d46 = ( 24.676 / 2 ) * 1 mm"
equation "d50 = ( ( 33.95 - 24.676 ) / 2 ) * 1 mm"
equation "d60 = 37.1 mm - 1.25 mm"
equation "d86 = ( 8.7 / 2 ) * 1 mm"
equation "d124 = ( 14.2 / 2 ) * 1 mm"
equation "d128 = ( 8.7 / 2 ) * 1 mm"
